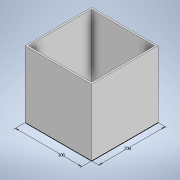
# Autodesk Inventor part: safe
Saved by Autodesk Inventor 2021 (Build 250183000, 183)
## iProperties
Created: 2021-05-19
Part Number: safe
Material: 일반
Document SubType Name: Modeling
Designer: Dongyoon
Density: 1 g/cm^3
Appearance: 기본값
Author: Dongyoon
Autodesk Inventor part; units mm, degrees
ref_plane "YZ Plane" through (0, 0, 0) normal (1, 0, 0) x (0, 1, 0)
ref_plane "XZ Plane" through (0, 0, 0) normal (0, 1, 0) x (-1, 0, 0)
ref_plane "XY Plane" through (0, 0, 0) normal (0, 0, 1) x (1, 0, 0)
sketch "스케치1" plane through (0, 0, 0) normal (0, 1, 0) x (-1, 0, 0)
  line L0 (100, -100) -> (-100, -100)
  line L1 (-100, -100) -> (-100, 100)
  line L2 (-100, 100) -> (100, 100)
  line L3 (100, 100) -> (100, -100)
  line L4 (100, -100) -> (-100, 100) construction
  line L5 (-100, -100) -> (100, 100) construction
  point P0 (0, 0)
  dimension "d0" = 200
  dimension "d1" = 200
  constraints: 12 end point, 2 midpoint, 2 parallel, 1 horizontal, 1 perpendicular
  measures "d0" distance of L1.end L2.end
  measures "d1" distance of L0.end L1.end
extrude "돌출1" add sketch "스케치1" along normal blind 200
sketch "스케치2" plane through (0, 200, 0) normal (0, 1, 0) x (1, 0, 0)
  line L0 (-95, 95) -> (95, 95)
  line L1 (95, 95) -> (95, -95)
  line L2 (95, -95) -> (-95, -95)
  line L3 (-95, -95) -> (-95, 95)
  line L4 (-95, 95) -> (95, -95) construction
  line L5 (95, 95) -> (-95, -95) construction
  point P0 (0, 0)
  dimension "d4" = 190
  dimension "d5" = 190
  constraints: 12 end point, 2 midpoint, 2 parallel, 1 horizontal, 1 perpendicular
  measures "d4" distance of L0.start L0.end
  measures "d5" distance of L0.end L1.end
extrude "돌출2" cut sketch "스케치2" against normal blind 195
